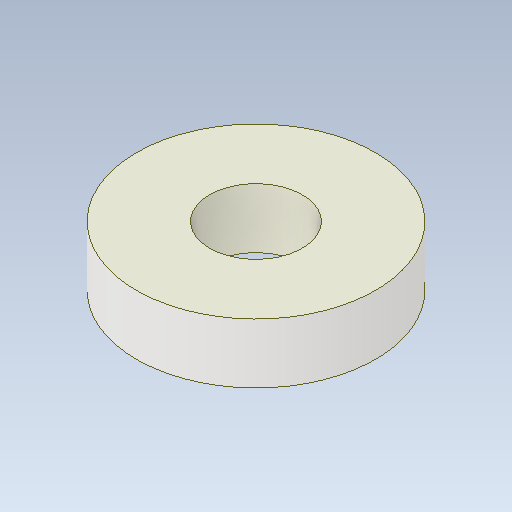
# Autodesk Inventor part: 275-1066
Saved by Autodesk Inventor 2020.2 (Build 242310000, 310)
## iProperties
Created: 2016-05-09
Part Number: 275-1066
Material: Glass
Document SubType Name: Modeling
Designer: Jacob
Density: 2.18 g/cm^3
Appearance: VEX Nylon
Author: Jacob (7842)
Autodesk Inventor part; units mm, degrees
ref_plane "YZ Plane" through (0, 0, 0) normal (1, 0, 0) x (0, 1, 0)
ref_plane "XZ Plane" through (0, 0, 0) normal (0, 1, 0) x (-1, 0, 0)
ref_plane "XY Plane" through (0, 0, 0) normal (0, 0, 1) x (1, 0, 0)
sketch "Sketch1" plane through (0, 0, 0) normal (0, 1, 0) x (-1, 0, 0)
  circle A0 centre (0, 0) radius 6.35
  circle A1 centre (0, 0) radius 2.4638
  dimension "d0" = 12.7
  dimension "d1" = 4.9276
  constraints: 2 centre point, 2 coincident
  measures "d0" diameter of A0
  measures "d1" diameter of A1
extrude "Extrusion1" add sketch "Sketch1" along normal blind 3.175
body "Solid1"
